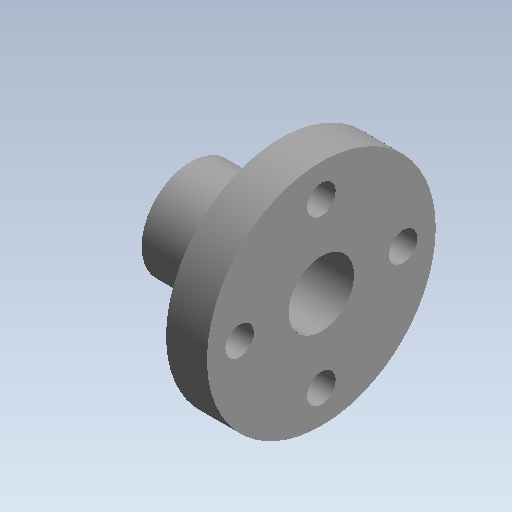
# Autodesk Inventor part: STHRB8_b
Saved by Autodesk Inventor 2020 (Build 240168000, 168)
## iProperties
Part Number: STHRB8_b
Material: Generic
Catalog Web Link: www.cadenas.de
Description: STHRB, STHR, SSTHR, ATHR, BTHR_b-Shaft Supports - Bracket Shaped - Standard Drilled Mounting Hole Type - Round Flange
Vendor: MISUMI
Document SubType Name: Modeling
Designer: partserver
Manufacturer: MISUMI
Mass: 3.3066 g
Surface Area: 25.408 cm^2
Volume: 3.3066 cm^3
Density: 1 g/cm^3
Appearance: PSOLRGB-192-192-192
Category: PARTsolutions
Company: MISUMI
PSOL_IDENT_0: {$CADENAS_DATA\23d-libs\misumi\metric\02_shaft_supports\ssthr\ssthr_body.prj},192 {VTYP=3D},{NB=STHR
PSOL_IDENT_1: B8_b},{LINA=STHRB8},{NN=STHRB, STHR, SSTHR, ATHR, BTHR_b},{DATE=30.03.2018 01:12:55},{GEOMDATE=06.10
PSOL_IDENT_2: .2015 08:50:00},{VERSION=},{LINEID=50},{WBVAR=MAT,ST,M,ALT},{WBNUMERIC=}  {NB=STHRB8_b},{LINA=STHRB8
PSOL_IDENT_3: },{KT=DUMMY},{PN=STHRB8},{TS=1},{TSALG= '1', 'Drilled Mounting Hole', '2', 'Tapped Mounting Hole' },
PSOL_IDENT_4: {TYPE=STHRB},{MAT=1018},{MATA= '1018', 'SS400 Equivalent', '304', 'SUS304', 'AA'  , 'Aluminum Alloy'
PSOL_IDENT_5: },{MALG='M3','M4'},{ST=BO},{ST0= 'BO', 'Black Oxide', 'ENP', 'Electroless Nickel Plating' },{D=8},{
PSOL_IDENT_6: THMD11='M3','M4'},{THMD13='M4'},{THMD12='M3'},{DTOL=+0.015/0},{DX=8},{N=2.0},{L=16},{D1=12},{H=28},{
PSOL_IDENT_7: T=5.0},{LL=10},{M=M3},{THMD=3},{THMD1=M3,M4},{THMD2=M3,M4},{P=20},{K=22},{W=16},{P1=20},{F=0},{DD1=3
PSOL_IDENT_8: .5},{DD11=3.5,4.5},{DD12=3.5,4.5},{M1=-},{M11=0},{ALT=},{ALTPN=},{BM=3.0},{BL=3.0}
NB: STHRB8_b
NN: STHRB, STHR, SSTHR, ATHR, BTHR_b
NT: Shaft Supports - Bracket Shaped - Standard Drilled Mounting Hole Type - Round Flange
NBSYN: $PN._b
LINA: STHRB8
CATALOG: Misumi
PN: STHRB8
MAT: SS400 Equivalent
ST: Black Oxide
D: 8
DTOL: +0.015/0
N: 2
L: 16
D1: 12
H: 28
T: 5
LL: 10
M: M3
P: 20
DD1: 3.5
ALT: w/o MB (Hex Socket Set Screw Included)
SUPPLIER: MISUMI
ARTICLENO: STHRB8_b
BOMINFO: STHRB8
CREATOR: CADENAS GmbH
Title: STHRB8
Author: Cadenas PARTsolutions
Comments: Shaft Supports - Bracket Shaped - Standard Drilled Mounting Hole Type - Round Flange
Autodesk Inventor part; units mm, degrees
ref_plane "YZ Plane" through (0, 0, 0) normal (1, 0, 0) x (0, 1, 0)
ref_plane "XZ Plane" through (0, 0, 0) normal (0, 1, 0) x (-1, 0, 0)
ref_plane "XY Plane" through (0, 0, 0) normal (0, 0, 1) x (1, 0, 0)
sketch "Sketch_1" plane through (0, 0, 0) normal (0, 0, 1) x (1, 0, 0)
  line L0 (16, 0) -> (0, 0)
  line L1 (0, 4) -> (16, 4)
  line L2 (16, 4) -> (16, 6)
  line L3 (16, 6) -> (5, 6)
  line L4 (5, 6) -> (5, 14)
  line L5 (5, 14) -> (0, 14)
  line L6 (0, 14) -> (0, 4)
  constraints: 14 end point
revolve "Revolution1" add sketch "Sketch_1" angle 360 about axis through (16, 0, 0) along (1, 0, 0)
sketch "Sketch_3" plane through (0, 0, 0) normal (0, -0.7071, 0.7071) x (1, 0, 0)
  line L0 (10, 3.5) -> (10, 6)
  line L1 (10, 6) -> (11.5, 6)
  line L2 (11.5, 6) -> (11.2295, 5.7295)
  line L3 (11.2295, 5.7295) -> (11.2295, 3.5)
  line L4 (11.2295, 3.5) -> (10, 3.5)
  line L5 (10, 3.5) -> (10, 6)
  constraints: 12 end point
revolve "Revolution2" cut sketch "Sketch_3" angle 360 about axis through (10, 2.4749, 2.4749) along (0, -0.7071, -0.7071)
thread "Thread1" size "M3x0.5" class "6H" standard "ISO Metric profile" length 2.2295
sketch "Sketch3" plane through (5, 0, 0) normal (1, 0, 0) x (0, 0, -1)
  point P0 (0, 10)
hole "Hole1" at (5, 10, 0) direction (-1, 0, 0) diameter 3.5 depth 5
sketch "Sketch4" plane through (5, 0, 0) normal (1, 0, 0) x (0, 0, -1)
  point P0 (0, -10)
hole "Hole2" at (5, -10, 0) direction (-1, 0, 0) diameter 3.5 depth 5
sketch "Sketch5" plane through (5, 0, 0) normal (1, 0, 0) x (0, 0, -1)
  point P0 (-10, 0)
hole "Hole3" at (5, 0, 10) direction (-1, 0, 0) diameter 3.5 depth 5
sketch "Sketch6" plane through (5, 0, 0) normal (1, 0, 0) x (0, 0, -1)
  point P0 (10, 0)
hole "Hole4" at (5, 0, -10) direction (-1, 0, 0) diameter 3.5 depth 5
sketch "Sketch_2" plane through (0, 0, 0) normal (0, -0.7071, -0.7071) x (1, 0, 0)
  line L0 (10, 3.5) -> (10, 6)
  line L1 (10, 6) -> (11.5, 6)
  line L2 (11.5, 6) -> (11.2295, 5.7295)
  line L3 (11.2295, 5.7295) -> (11.2295, 3.5)
  line L4 (11.2295, 3.5) -> (10, 3.5)
  line L5 (10, 3.5) -> (10, 6)
  constraints: 12 end point
revolve "Revolution3" cut sketch "Sketch_2" angle 360 about axis through (10, -2.4749, 2.4749) along (0, 0.7071, -0.7071)
thread "Thread2" size "M3x0.5" class "6H" standard "ISO Metric profile" length 2.2295
body "Solid1"
